Axe 4 (Autodesk Fusion 360 design; units mm, degrees)
Autodesk Fusion 360 part; units mm, degrees
sketch "Sketch1" plane through (0, 0, 0) normal (0, 0, 1) x (1, 0, 0)
  circle A0 centre (0, 0) radius 9
  circle A1 centre (0, 0) radius 6 construction
  circle A2 centre (-0.0008, 6) radius 2
  circle A3 centre (-6, -0.0008) radius 2
  circle A4 centre (0.0008, -6) radius 2
  circle A5 centre (6, 0.0008) radius 2
  circle A6 centre (0, 0) radius 2.1
  dimension "d1" = 18
  dimension "d2" = 12
  dimension "d3" = 4
  dimension "d5" = 360
  dimension "d25" = 4.2
  constraint coincident A0.centre A1.centre
  constraint concentric A0 A1
  constraint coincident A1 A2.centre
  constraint concentric A0 A6
  measures "d1" diameter of A0
  measures "d2" diameter of A1
  measures "d3" diameter of A2
  measures "d25" diameter of A6
extrude "Extrude1" add sketch "Sketch1" against normal blind 4 contours A0 | A2 | A3 | A4 | A5
extrude "Extrude2" add sketch "Sketch1" along normal blind 3 contours A2 | A3 | A4 | A5
sketch "Sketch7" plane through (0, 0, 0) normal (0, 0, 1) x (-1, 0, 0)
  circle A0 centre (-6, -0.0008) radius 2
  circle A1 centre (6, 0.0008) radius 2
  circle A2 centre (0.0008, -6) radius 2
  circle A3 centre (-0.0008, 6) radius 2
  circle A4 centre (0, 0) radius 2.1
  circle A5 centre (0, 0) radius 9
  line L0 (-4.1569, 0) -> (-2.0785, -3.6)
  line L1 (-2.0785, -3.6) -> (2.0785, -3.6)
  line L2 (2.0785, -3.6) -> (4.1569, 0)
  line L3 (4.1569, 0) -> (2.0785, 3.6)
  line L4 (2.0785, 3.6) -> (-2.0785, 3.6)
  line L5 (-2.0785, 3.6) -> (-4.1569, 0)
  dimension "d26" = 7.2
  constraint coincident A4.centre A5.centre
  constraint horizontal L1
  measures "d26" distance of L1 L4
extrude "Extrude8" cut sketch "Sketch7" against normal blind 2.5 contours A0 L0 L5 | A0 A1 L0 L1 L2 L3 L4 L5 | A1 L2 L3 picked at (-4.0529, 0.0269) picked at (4.0534, 0.0001)
named bodies: "Axe4"
